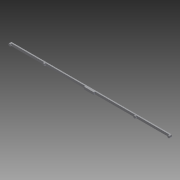
# Autodesk Inventor part: connection2
Saved by Autodesk Inventor 2011 (Build 150239000, 239)
## iProperties
Created: 2011-07-10
Part Number: connection2
Document SubType Name: Modeling
Designer: adowning
Density: 1 g/cm^3
Author: adowning
Autodesk Inventor part; units mm, degrees
ref_plane "YZ Plane" through (0, 0, 0) normal (1, 0, 0) x (0, 1, 0)
ref_plane "XZ Plane" through (0, 0, 0) normal (0, 1, 0) x (-1, 0, 0)
ref_plane "XY Plane" through (0, 0, 0) normal (0, 0, 1) x (1, 0, 0)
sketch "Sketch1" plane through (0, 0, 0) normal (0, 0, 1) x (1, 0, 0)
  line L0 (-44.0493, 3.2293) -> (375.8381, 3.2293)
  line L1 (375.8381, 3.2293) -> (375.8381, -3.1207)
  line L2 (375.8381, -3.1207) -> (-44.0493, -3.1207)
  line L3 (-44.0493, -3.1207) -> (-44.0493, 3.2293)
  circle A0 centre (-44.0493, 0.0543) radius 3.175
  circle A1 centre (375.8381, 0.0543) radius 3.175
  point P0 (0, 0)
  dimension "d0" = 419.8874
  dimension "d1" = 6.35
  constraints: 8 end point, 2 midpoint, 2 parallel, 1 centre point, 1 horizontal, 1 perpendicular, 1 tangent, 1 vertical alignment, 2 other
  measures "d0" distance of L1.end L2.end
  measures "d1" distance of L0.end L1.end
extrude "Extrusion1" add sketch "Sketch1" along normal blind 3.175
sketch "Sketch2" plane through (0, 0, 3.175) normal (0, 0, 1) x (1, 0, 0)
  arc A0 (375.8381, -3.1207) -> (375.8381, 3.2293) centre (375.8381, 0.0543) ccw projected
  line L0 (-44.0493, 3.2293) -> (375.8381, 3.2293) projected
  arc A1 (-44.0493, 3.2293) -> (-44.0493, -3.1207) centre (-44.0493, 0.0543) ccw projected
  line L1 (375.8381, -3.1207) -> (-44.0493, -3.1207) projected
  circle A2 centre (-44.0493, 0.0543) radius 3.175
  circle A3 centre (375.8381, 0.0543) radius 3.175
  line L2 (-44.0493, 0.0543) -> (45.6381, 0.0543)
  circle A4 centre (45.6381, 0.0543) radius 3.175
  line L3 (375.8381, 0.0543) -> (286.1507, 0.0543)
  circle A5 centre (286.1507, 0.0543) radius 3.175
  line L4 (45.6381, 0.0543) -> (286.1507, 0.0543)
  line L5 (45.6381, 3.2293) -> (286.1507, -3.1207)
  line L6 (165.8944, 0.0543) -> (165.8944, -3.1207)
  line L7 (165.8944, -3.1207) -> (153.1944, -3.1207)
  line L8 (153.1944, -3.1207) -> (178.5944, -3.1207)
  line L9 (178.5944, -3.1207) -> (178.5944, 3.2293)
  line L10 (178.5944, 3.2293) -> (153.1944, 3.2293)
  line L11 (153.1944, 3.2293) -> (153.1944, -3.1207)
  point P0 (0, 0)
  dimension "d4" = 89.6874
  dimension "d5" = 89.6874
  dimension "d6" = 12.7
  dimension "d7" = 25.4
  constraints: 20 end point, 4 coincident, 4 point on line, 3 horizontal, 3 parallel, 2 centre point, 2 collinear, 2 midpoint, 2 vertical alignment, 1 concentric, 1 perpendicular, 1 tangent, 4 other
  measures "d4" distance of L2.start L2.end
  measures "d5" distance of L3.start L3.end
  measures "d6" distance of L6.end L7.end
  measures "d7" distance of L10.end L9.end
extrude "Extrusion2" add sketch "Sketch2" along normal blind 3.175 contours A3 A0 | A5 L4 L3 | L1 L6 L5 L9 | L3 L4 A5 | L5 L4 L9 | L1 L11 L4 L6 | L4 L5 L11 L0 L9 | L4 L11 L5 | A4 L4 L2 | A4 L2 L4 | A1 A2
body "Solid1"
